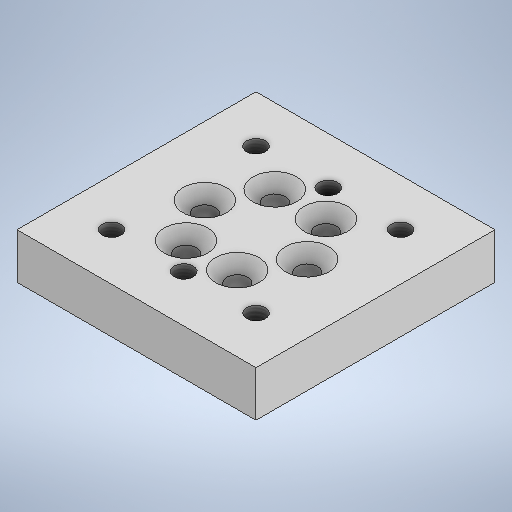
# Autodesk Inventor part: Adapter plate for tube dovetail bracket
Saved by Autodesk Inventor 2025 (Build 290162000, 162)
## iProperties
Created: 2025-08-12
Part Number: Adapter plate for tube dovetail bracket
Material: Generic
Document SubType Name: Modeling
Designer: yshis
Density: 1 g/cm^3
Appearance: Default
Author: yshis
Autodesk Inventor part; units mm, degrees
ref_plane "YZ Plane" through (0, 0, 0) normal (1, 0, 0) x (0, 1, 0)
ref_plane "XZ Plane" through (0, 0, 0) normal (0, 1, 0) x (-1, 0, 0)
ref_plane "XY Plane" through (0, 0, 0) normal (0, 0, 1) x (1, 0, 0)
sketch "Sketch1" plane through (0, 0, 0) normal (0, 1, 0) x (-1, 0, 0)
  line L0 (0, 0) -> (63, 0)
  line L1 (63, 0) -> (63, -63)
  line L2 (63, -63) -> (0, -63)
  line L3 (0, -63) -> (0, 0)
  circle A0 centre (31.5, -31.5) radius 3.1
  circle A1 centre (12.45, -12.45) radius 2.5
  circle A2 centre (31.5, -12.45) radius 2.5
  circle A3 centre (50.55, -12.45) radius 2.5
  circle A4 centre (12.45, -50.55) radius 2.5
  circle A5 centre (31.5, -50.55) radius 2.5
  circle A6 centre (50.55, -50.55) radius 2.5
  point P0 (31.5, -63)
  dimension "d0" = 63
  dimension "d1" = 63
  dimension "d2" = 6.2
  dimension "d3" = 31.5
  dimension "d4" = 31.5
  dimension "d5" = 19.05
  dimension "d6" = 19.05
  dimension "d7" = 5
  dimension "d10" = 19.05
  dimension "d13" = 38.1
  constraints: 8 end point, 7 centre point, 2 horizontal, 2 parallel, 1 midpoint, 1 perpendicular, 1 vertical, 10 other
  measures "d0" distance of L1.end L2.end
  measures "d1" distance of L0.end L1.end
  measures "d2" diameter of A0
  measures "d3" distance of point (31.5, -63) A0.centre
  measures "d4" distance from line of A0.centre L3
  measures "d5" horizontal distance of A1.centre A0.centre
  measures "d6" horizontal distance of A1.centre A0.centre
  measures "d7" diameter of A1
  measures "d10" distance of A1.centre A2.centre
  measures "d13" distance of A1.centre A4.centre
extrude "Extrusion1" add sketch "Sketch1" along normal blind 12 contours L0 L1 L2 L3 | A0
sketch "Sketch2" plane through (0, 12, 0) normal (0, 1, 0) x (1, 0, 0)
  circle A0 centre (-45, 31.5) radius 2.75
  circle A1 centre (-31.5, 31.5) radius 3.1 projected
  circle A2 centre (-38.25, 19.8087) radius 2.75
  circle A3 centre (-24.75, 19.8087) radius 2.75
  circle A4 centre (-18, 31.5) radius 2.75
  circle A5 centre (-24.75, 43.1913) radius 2.75
  circle A6 centre (-38.25, 43.1913) radius 2.75
  point P0 (0, 0)
  dimension "d18" = 5.5
  dimension "d19" = 13.5
  dimension "d20" = 0
  dimension "d23" = 360
  constraints: 6 centre point, 13 other
  measures "d18" diameter of A0
  measures "d19" distance of A1.centre A0.centre
  measures "d20" vertical distance of A0.centre A1.centre
extrude "Extrusion2" cut sketch "Sketch2" against normal blind 12 contours A0 | A2 | A3 | A4 | A5 | A6
chamfer "Chamfer1" distance 3 angle 45 6 edges at (-41, 12, -43.1913) (-47.75, 12, -31.5) (-41, 12, -19.8087) (-27.5, 12, -19.8087) (-20.75, 12, -31.5) (-27.5, 12, -43.1913)
thread "Thread2" size "M6x1" class "6H" standard "ANSI Metric M Profile" full length
thread "Thread3" size "M5x0.8" class "6H" standard "ANSI Metric M Profile" full length
thread "Thread4" size "M5x0.8" class "6H" standard "ANSI Metric M Profile" full length
thread "Thread5" size "M5x0.8" class "6H" standard "ANSI Metric M Profile" full length
thread "Thread6" size "M5x0.8" class "6H" standard "ANSI Metric M Profile" full length
thread "Thread7" size "M5x0.8" class "6H" standard "ANSI Metric M Profile" full length
equation "\"d3\" = 0.5 * d1"
equation "\"d4\" = 0.5 * d0"
body "Solid1"
